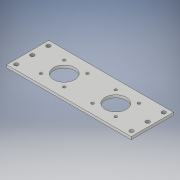
# Autodesk Inventor part: 3D Camera Mount 3
Saved by Autodesk Inventor 2017 (Build 210142000, 142)
## iProperties
Created: 2016-10-01
Part Number: 3D Camera Mount 3
Material: Generic
Document SubType Name: Modeling
Designer: Sofia
Density: 1 g/cm^3
Appearance: Default
Author: Sofia
Autodesk Inventor part; units mm, degrees
ref_plane "YZ Plane" through (0, 0, 0) normal (1, 0, 0) x (0, 1, 0)
ref_plane "XZ Plane" through (0, 0, 0) normal (0, 1, 0) x (-1, 0, 0)
ref_plane "XY Plane" through (0, 0, 0) normal (0, 0, 1) x (1, 0, 0)
sketch "Sketch1" plane through (0, 0, 0) normal (0, 1, 0) x (-1, 0, 0)
  line L0 (0, 0) -> (-149.86, 0)
  line L1 (-149.86, 0) -> (-149.86, -50.8)
  line L2 (-149.86, -50.8) -> (0, -50.8)
  line L3 (0, -50.8) -> (0, 0)
  circle A0 centre (-43.942, -25.4) radius 12.7
  circle A1 centre (-29.972, -39.37) radius 1.5875
  circle A2 centre (-57.912, -39.37) radius 1.5875
  circle A3 centre (-57.912, -11.43) radius 1.5875
  circle A4 centre (-29.972, -11.43) radius 1.5875
  line L4 (-74.93, -50.8) -> (-74.93, 0) construction
  circle A5 centre (-5.588, -44.704) radius 2.3495
  circle A6 centre (-5.588, -25.4) radius 2.3495
  circle A7 centre (-5.588, -6.096) radius 2.3495
  circle A8 centre (-105.918, -25.4) radius 12.7
  circle A9 centre (-119.888, -39.37) radius 1.5875
  circle A10 centre (-91.948, -39.37) radius 1.5875
  circle A11 centre (-91.948, -11.43) radius 1.5875
  circle A12 centre (-119.888, -11.43) radius 1.5875
  circle A13 centre (-144.272, -44.704) radius 2.3495
  circle A14 centre (-144.272, -25.4) radius 2.3495
  circle A15 centre (-144.272, -6.096) radius 2.3495
  point P0 (-74.93, -25.4)
  dimension "d0" = 149.86
  dimension "d1" = 50.8
  dimension "d2" = 30.988
  dimension "d3" = 25.4
  dimension "d4" = 25.4
  dimension "d5" = 13.97
  dimension "d6" = 13.97
  dimension "d7" = 13.97
  dimension "d8" = 13.97
  dimension "d9" = 13.97
  dimension "d10" = 13.97
  dimension "d11" = 13.97
  dimension "d12" = 13.97
  dimension "d13" = 3.175
  dimension "d14" = 3.175
  dimension "d15" = 3.175
  dimension "d16" = 3.175
  dimension "d17" = 5.588
  dimension "d18" = 6.096
  dimension "d19" = 5.588
  dimension "d20" = 25.4
  dimension "d21" = 6.096
  dimension "d22" = 5.588
  dimension "d23" = 4.699
  dimension "d24" = 4.699
  dimension "d25" = 4.699
  constraints: 16 centre point, 12 coincident, 12 symmetric about line, 10 end point, 2 midpoint, 2 parallel, 1 horizontal, 1 perpendicular, 8 other
  measures "d0" distance of L2.end L1.end
  measures "d1" distance of L1.end L0.end
  measures "d2" distance of point (-43.942, -25.4) point (-74.93, -25.4)
  measures "d3" distance from line of L2 point (-43.942, -25.4)
  measures "d4" diameter of A0
  measures "d5" horizontal distance of point (-57.912, -39.37) A0.centre
  measures "d6" horizontal distance of point (-57.912, -39.37) point (-43.942, -25.4)
  measures "d7" horizontal distance of point (-57.912, -11.43) point (-43.942, -25.4)
  measures "d8" horizontal distance of point (-57.912, -11.43) point (-43.942, -25.4)
  measures "d9" horizontal distance of point (-43.942, -25.4) point (-29.972, -11.43)
  measures "d10" horizontal distance of point (-29.972, -11.43) point (-43.942, -25.4)
  measures "d11" horizontal distance of point (-29.972, -39.37) point (-43.942, -25.4)
  measures "d12" horizontal distance of point (-43.942, -25.4) point (-29.972, -39.37)
  measures "d13" diameter of A1
  measures "d14" diameter of A2
  measures "d15" diameter of A3
  measures "d16" diameter of A4
  measures "d17" distance from line of L3 point (-5.588, -44.704)
  measures "d18" distance from line of L2 point (-5.588, -44.704)
  measures "d19" distance from line of L3 point (-5.588, -25.4)
  measures "d20" vertical distance of L0.start point (-5.588, -25.4)
  measures "d21" distance from line of point (-5.588, -6.096) L0
  measures "d22" distance from line of L3 point (-5.588, -6.096)
  measures "d23" diameter of A5
  measures "d24" diameter of A6
  measures "d25" diameter of A7
extrude "Extrusion1" add sketch "Sketch1" along normal blind 3.175
body "Solid1"
